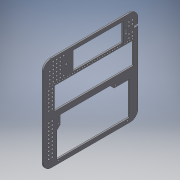
# Autodesk Inventor part: TrayPanelB
Saved by Autodesk Inventor 2017 (Build 210142000, 142)
## iProperties
Created: 2019-06-22
Part Number: TrayPanelB
Material: Generic
Document SubType Name: Modeling
Designer: DDeGo
Density: 1 g/cm^3
Appearance: Default
Author: DDeGo
Autodesk Inventor part; units mm, degrees
ref_plane "YZ Plane" through (0, 0, 0) normal (1, 0, 0) x (0, 1, 0)
ref_plane "XZ Plane" through (0, 0, 0) normal (0, 1, 0) x (-1, 0, 0)
ref_plane "XY Plane" through (0, 0, 0) normal (0, 0, 1) x (1, 0, 0)
sketch "Block1" plane through (0, 0, 0) normal (0, 0, 1) x (1, 0, 0)
  circle A0 centre (31, 19.5) radius 1.5
  line L0 (34, 5.5) -> (34, 22.5)
  line L1 (34, 22.5) -> (27, 29.5)
  line L2 (27, 29.5) -> (27, 80.5)
  circle A1 centre (31, 83.5) radius 1.5
  line L3 (134, 5.5) -> (34, 5.5)
  line L4 (173, 80.5) -> (173, 13.5)
  circle A2 centre (169, 83.5) radius 1.5
  line L5 (27, 80.5) -> (173, 80.5)
  line L6 (173, 13.5) -> (142, 13.5)
  line L7 (142, 13.5) -> (134, 5.5)
  circle A3 centre (145, 9.5) radius 1.5
  point P0 (93.25, 35.7812)
sketch "Sketch1" plane through (0, 0, 0) normal (1, 0, 0) x (0, 1, 0)
  line L0 (59.5116, 142.721) -> (59.5116, 146.221) construction
  line L1 (59.5116, 182.721) -> (159.5116, 182.721)
  line L2 (159.5116, 182.721) -> (159.5116, 142.721)
  line L3 (159.5116, 142.721) -> (158.0116, 142.721)
  line L4 (21.5116, 95.221) -> (21.5116, 139.921)
  line L5 (21.5116, 139.921) -> (180.5116, 139.921)
  line L6 (180.5116, 139.921) -> (180.5116, 95.221)
  line L7 (180.5116, 95.221) -> (21.5116, 95.221)
  line L8 (174.0116, 190.221) -> (15.0116, 190.221)
  arc A0 (15.0116, 190.221) -> (-0.4884, 174.721) centre (15.0116, 174.721) ccw
  line L9 (-0.4884, 174.721) -> (-0.4884, 15.721)
  arc A1 (-0.4884, 15.721) -> (15.0116, 0.221) centre (15.0116, 15.721) ccw
  line L10 (15.0116, 0.221) -> (174.0116, 0.221)
  arc A2 (174.0116, 0.221) -> (189.5116, 15.721) centre (174.0116, 15.721) ccw
  line L11 (189.5116, 15.721) -> (189.5116, 174.721)
  arc A3 (189.5116, 174.721) -> (174.0116, 190.221) centre (174.0116, 174.721) ccw
  line L12 (158.0116, 142.721) -> (158.0116, 146.221)
  line L13 (158.0116, 146.221) -> (59.5116, 146.221)
  line L14 (158.0116, 142.721) -> (59.5116, 142.721) construction
  line L15 (59.5116, 146.221) -> (59.5116, 182.721)
  circle A4 centre (30.5116, 69.721) radius 1.5
  line L16 (33.5116, 83.721) -> (33.5116, 66.721)
  line L17 (33.5116, 66.721) -> (26.5116, 59.721)
  line L18 (26.5116, 59.721) -> (26.5116, 8.721)
  circle A5 centre (30.5116, 5.721) radius 1.5
  line L19 (133.5116, 83.721) -> (33.5116, 83.721)
  line L20 (172.5116, 8.721) -> (172.5116, 75.721)
  circle A6 centre (168.5116, 5.721) radius 1.5
  line L21 (26.5116, 8.721) -> (172.5116, 8.721)
  line L22 (172.5116, 75.721) -> (141.5116, 75.721)
  line L23 (141.5116, 75.721) -> (133.5116, 83.721)
  circle A7 centre (144.5116, 79.721) radius 1.5
  dimension "d2" = 100
  dimension "d4" = 190
  dimension "d5" = 190
  dimension "d8" = 95
  dimension "d10" = 22
  dimension "d11" = 60
  dimension "d12" = 44.7
  dimension "d13" = 159
  dimension "d14" = 15.5
  dimension "d47" = 5.5
  dimension "d48" = 27
  dimension "d65" = 3.5
  dimension "d66" = 1.5
  dimension "d67" = 146
  dimension "d68" = 36.5
  constraints: 32 end point, 8 point on circle, 8 tangent, 4 centre point, 4 horizontal, 4 vertical, 3 equal radius, 2 perpendicular, 1 other
  measures "d2" distance between parallel lines of L0 L2
  measures "d4" distance between parallel lines of L11 L9
  measures "d5" distance between parallel lines of L8 L10
  measures "d8" distance between parallel lines of L10 L7
  measures "d10" distance between parallel lines of L4 L9
  measures "d11" distance between parallel lines of L0 L9
  measures "d12" distance between parallel lines of L5 L7
  measures "d13" distance between parallel lines of L4 L6
  measures "d14" radius of A0
  measures "d65" distance between parallel lines of L3 L13
  measures "d66" distance between parallel lines of L2 L12
  measures "d67" distance between parallel lines of L10 L13
  measures "d68" distance between parallel lines of L1 L13
extrude "Extrusion1" add sketch "Sketch1" along normal blind 2.75
sketch "Sketch2" plane through (2.75, 0, 0) normal (1, 0, 0) x (0, 0, -1)
  circle A0 centre (-148.221, 54.5116) radius 2
  line L0 (-142.721, 159.5116) -> (-142.721, 158.0116) projected
  line L1 (-146.221, 59.5116) -> (-179.9149, 59.5116) construction
  circle A1 centre (-148.221, 47.5116) radius 2
  circle A2 centre (-148.221, 40.5116) radius 2
  circle A3 centre (-148.221, 33.5116) radius 2
  circle A4 centre (-148.221, 26.5116) radius 2
  circle A5 centre (-148.221, 19.5116) radius 2
  circle A6 centre (-148.221, 12.5116) radius 2
  circle A7 centre (-155.221, 54.5116) radius 2
  circle A8 centre (-155.221, 47.5116) radius 2
  circle A9 centre (-155.221, 40.5116) radius 2
  circle A10 centre (-155.221, 33.5116) radius 2
  circle A11 centre (-155.221, 26.5116) radius 2
  circle A12 centre (-155.221, 19.5116) radius 2
  circle A13 centre (-155.221, 12.5116) radius 2
  circle A14 centre (-162.221, 54.5116) radius 2
  circle A15 centre (-162.221, 47.5116) radius 2
  circle A16 centre (-162.221, 40.5116) radius 2
  circle A17 centre (-162.221, 33.5116) radius 2
  circle A18 centre (-162.221, 26.5116) radius 2
  circle A19 centre (-162.221, 19.5116) radius 2
  circle A20 centre (-162.221, 12.5116) radius 2
  circle A21 centre (-169.221, 54.5116) radius 2
  circle A22 centre (-169.221, 47.5116) radius 2
  circle A23 centre (-169.221, 40.5116) radius 2
  circle A24 centre (-169.221, 33.5116) radius 2
  circle A25 centre (-169.221, 26.5116) radius 2
  circle A26 centre (-169.221, 19.5116) radius 2
  circle A27 centre (-169.221, 12.5116) radius 2
  circle A28 centre (-176.221, 54.5116) radius 2
  circle A29 centre (-176.221, 47.5116) radius 2
  circle A30 centre (-176.221, 40.5116) radius 2
  circle A31 centre (-176.221, 33.5116) radius 2
  circle A32 centre (-176.221, 26.5116) radius 2
  circle A33 centre (-176.221, 19.5116) radius 2
  circle A34 centre (-176.221, 12.5116) radius 2
  circle A35 centre (-183.221, 54.5116) radius 2
  circle A36 centre (-183.221, 47.5116) radius 2
  circle A37 centre (-183.221, 40.5116) radius 2
  circle A38 centre (-183.221, 33.5116) radius 2
  circle A39 centre (-183.221, 26.5116) radius 2
  circle A40 centre (-183.221, 19.5116) radius 2
  circle A41 centre (-183.221, 12.5116) radius 2
  line L2 (-148.221, 54.5116) -> (-148.221, 164.5116) construction
  circle A42 centre (-148.221, 164.5116) radius 2
  line L3 (-182.721, 159.5116) -> (-142.721, 159.5116) projected
  circle A43 centre (-148.221, 171.5116) radius 2
  circle A44 centre (-148.221, 178.5116) radius 2
  circle A45 centre (-155.221, 164.5116) radius 2
  circle A46 centre (-155.221, 171.5116) radius 2
  circle A47 centre (-155.221, 178.5116) radius 2
  circle A48 centre (-162.221, 164.5116) radius 2
  circle A49 centre (-162.221, 171.5116) radius 2
  circle A50 centre (-162.221, 178.5116) radius 2
  circle A51 centre (-169.221, 164.5116) radius 2
  circle A52 centre (-169.221, 171.5116) radius 2
  circle A53 centre (-169.221, 178.5116) radius 2
  circle A54 centre (-176.221, 164.5116) radius 2
  circle A55 centre (-176.221, 171.5116) radius 2
  circle A56 centre (-176.221, 178.5116) radius 2
  circle A57 centre (-183.221, 164.5116) radius 2
  circle A58 centre (-183.221, 171.5116) radius 2
  circle A59 centre (-183.221, 178.5116) radius 2
  circle A60 centre (-143.071, 12.5116) radius 1.5
  line L4 (-139.921, 21.5116) -> (-139.921, 180.5116) projected
  line L5 (-139.921, 12.5116) -> (-143.071, 12.5116) construction
  line L6 (-143.071, 12.5116) -> (-146.221, 12.5116) construction
  line L7 (-146.221, 12.5116) -> (-148.221, 12.5116) construction
  circle A61 centre (-143.071, 17.5419) radius 1.5
  circle A62 centre (-143.071, 22.5722) radius 1.5
  circle A63 centre (-143.071, 27.6025) radius 1.5
  circle A64 centre (-143.071, 32.6328) radius 1.5
  circle A65 centre (-143.071, 37.6631) radius 1.5
  circle A66 centre (-143.071, 42.6934) radius 1.5
  circle A67 centre (-143.071, 47.7237) radius 1.5
  circle A68 centre (-143.071, 52.754) radius 1.5
  circle A69 centre (-143.071, 57.7843) radius 1.5
  circle A70 centre (-143.071, 62.8146) radius 1.5
  circle A71 centre (-143.071, 67.8449) radius 1.5
  circle A72 centre (-143.071, 72.8752) radius 1.5
  circle A73 centre (-143.071, 77.9055) radius 1.5
  circle A74 centre (-143.071, 82.9358) radius 1.5
  circle A75 centre (-143.071, 87.9661) radius 1.5
  circle A76 centre (-143.071, 92.9964) radius 1.5
  circle A77 centre (-143.071, 98.0267) radius 1.5
  circle A78 centre (-143.071, 103.057) radius 1.5
  circle A79 centre (-143.071, 108.0873) radius 1.5
  circle A80 centre (-143.071, 113.1176) radius 1.5
  circle A81 centre (-143.071, 118.1479) radius 1.5
  circle A82 centre (-143.071, 123.1782) radius 1.5
  circle A83 centre (-143.071, 128.2085) radius 1.5
  circle A84 centre (-143.071, 133.2388) radius 1.5
  circle A85 centre (-143.071, 138.2691) radius 1.5
  circle A86 centre (-143.071, 143.2994) radius 1.5
  circle A87 centre (-143.071, 148.3298) radius 1.5
  circle A88 centre (-143.071, 153.3601) radius 1.5
  circle A89 centre (-143.071, 158.3904) radius 1.5
  circle A90 centre (-143.071, 163.4207) radius 1.5
  circle A91 centre (-143.071, 168.451) radius 1.5
  circle A92 centre (-143.071, 173.4813) radius 1.5
  circle A93 centre (-143.071, 178.5116) radius 1.5
  line L8 (-148.221, 178.5116) -> (-143.071, 178.5116) construction
  line L9 (-146.221, 59.5116) -> (-182.721, 59.5116) construction
  line L10 (-146.221, 158.0116) -> (-146.221, 59.5116) projected
  circle A94 centre (-136.771, 10.5116) radius 2
  line L11 (-139.921, 12.5116) -> (-136.771, 12.5116) construction
  line L12 (-136.771, 12.5116) -> (-136.771, 10.5116) construction
  circle A95 centre (-136.771, 17.5116) radius 2
  circle A96 centre (-129.771, 10.5116) radius 2
  circle A97 centre (-129.771, 17.5116) radius 2
  circle A98 centre (-122.771, 10.5116) radius 2
  circle A99 centre (-122.771, 17.5116) radius 2
  circle A100 centre (-115.771, 10.5116) radius 2
  circle A101 centre (-115.771, 17.5116) radius 2
  circle A102 centre (-108.771, 10.5116) radius 2
  circle A103 centre (-108.771, 17.5116) radius 2
  circle A104 centre (-101.771, 10.5116) radius 2
  circle A105 centre (-101.771, 17.5116) radius 2
  circle A106 centre (-94.771, 10.5116) radius 2
  circle A107 centre (-94.771, 17.5116) radius 2
  circle A108 centre (-87.771, 10.5116) radius 2
  circle A109 centre (-87.771, 17.5116) radius 2
  circle A110 centre (-80.771, 10.5116) radius 2
  circle A111 centre (-80.771, 17.5116) radius 2
  circle A112 centre (-73.771, 10.5116) radius 2
  circle A113 centre (-73.771, 17.5116) radius 2
  circle A114 centre (-66.771, 10.5116) radius 2
  circle A115 centre (-66.771, 17.5116) radius 2
  circle A116 centre (-59.771, 10.5116) radius 2
  circle A117 centre (-59.771, 17.5116) radius 2
  circle A118 centre (-52.771, 10.5116) radius 2
  circle A119 centre (-52.771, 17.5116) radius 2
  circle A120 centre (-45.771, 10.5116) radius 2
  circle A121 centre (-45.771, 17.5116) radius 2
  circle A122 centre (-38.771, 10.5116) radius 2
  circle A123 centre (-38.771, 17.5116) radius 2
  circle A124 centre (-31.771, 10.5116) radius 2
  circle A125 centre (-31.771, 17.5116) radius 2
  circle A126 centre (-24.771, 10.5116) radius 2
  circle A127 centre (-24.771, 17.5116) radius 2
  circle A128 centre (-17.771, 10.5116) radius 2
  circle A129 centre (-17.771, 17.5116) radius 2
  point P0 (0, 0)
  dimension "d15" = 4
  dimension "d17" = 5
  dimension "d20" = 7
  dimension "d23" = 7
  dimension "d28" = 5
  dimension "d31" = 7
  dimension "d34" = 7
  dimension "d37" = 3
  dimension "d40" = 5.0303
  dimension "d69" = 2
  dimension "d77" = 7
  dimension "d80" = 7
  dimension "d83" = 2
  constraints: 129 centre point, 16 end point, 9 horizontal, 8 equal radius, 8 vertical alignment, 3 vertical, 2 collinear, 2 point on line, 1 coincident, 1 horizontal alignment, 1 perpendicular, 241 other
  measures "d15" diameter of A0
  measures "d17" distance from line of L2.start L1
  measures "d20" distance of L2.start A1.centre
  measures "d23" distance of L2.start A7.centre
  measures "d28" distance from line of L3 A42.centre
  measures "d31" distance of A42.centre A43.centre
  measures "d34" distance of A42.centre A45.centre
  measures "d37" diameter of A60
  measures "d40" distance of L5.end A61.centre
  measures "d69" distance between parallel lines of L10 L2
  measures "d77" distance of L12.end A95.centre
  measures "d80" distance of L12.end A96.centre
  measures "d83" distance of L11.end L12.end
extrude "Extrusion2" cut sketch "Sketch2" against normal blind 10 contours A3 | A4 | A5 | A6 | A10 | A11 | A12 | A13 | A17 | A18 | A19 | A20 | A24 | A25 | A26 | A27 | A31 | A32 | A33 | A38 | A39 | A40 | A43 | A44 | A46 | A47 | A52 | A53 | A55 | A56 | A60 | A61 | A62 | A63 | A64 | A65 | A66 | A67 | A68 | A69 | A70 | A71 | A72 | A73 | A74 | A75 | A76 | A77 | A78 | A79 | A80 | A81 | A82 | A83 | A84 | A85 | A86 | A87 | A88 | A90 | A91 | A92 | A93 | A94 | A95 | A96 | A97 | A98 | A99 | A100 | A101 | A102 | A103 | A104 | A105 | A110 | A111 | A112 | A113 | A114 | A115 | A116 | A117 | A118 | A119 | A120 | A121 | A122 | A123 | A124 | A125 | A126 | A127 | A128 | A129
sketch "Sketch3" plane through (0, 0, 0) normal (-1, 0, 0) x (0, 0, 1)
  line L0 (167.221, 168.2116) -> (157.221, 168.2116)
  line L1 (157.221, 168.2116) -> (157.221, 163.9116)
  line L2 (157.221, 163.9116) -> (167.221, 163.9116)
  line L3 (167.221, 163.9116) -> (167.221, 168.2116)
  line L4 (142.721, 158.0116) -> (142.721, 159.5116) projected
  line L5 (142.721, 159.5116) -> (182.721, 159.5116) projected
  line L6 (164.371, 189.5116) -> (160.071, 189.5116)
  line L7 (160.071, 189.5116) -> (160.071, 181.5116)
  line L8 (160.071, 181.5116) -> (164.371, 181.5116)
  line L9 (164.371, 181.5116) -> (164.371, 189.5116)
  line L10 (174.721, 189.5116) -> (15.721, 189.5116) projected
  line L11 (162.221, 181.5116) -> (162.221, 168.2116) construction
  point P0 (0, 0)
  point P1 (143.721, 59.5116)
  dimension "d49" = 4.3
  dimension "d50" = 10
  dimension "d51" = 14.5
  dimension "d52" = 4.4
  dimension "d55" = 4.3
  dimension "d56" = 8
  constraints: 18 end point, 4 parallel, 2 horizontal, 2 midpoint, 2 perpendicular, 1 point on line, 1 vertical, 1 other
  measures "d49" distance of L2.end L0.start
  measures "d50" distance of L1.end L2.end
  measures "d52" distance between parallel lines of L5 L2
  measures "d55" distance of L7.end L8.end
  measures "d56" distance between parallel lines of L6 L8
extrude "Extrusion3" cut sketch "Sketch3" against normal blind 10
sketch "Sketch4" plane through (0, 0, 0) normal (-1, 0, 0) x (0, 0, 1)
  circle A0 centre (179.721, 179.0116) radius 2.05
  line L0 (190.221, 15.0116) -> (190.221, 174.0116) projected
  line L1 (174.721, 189.5116) -> (164.371, 189.5116) projected
  circle A1 centre (10.721, 10.0116) radius 2.05
  line L2 (15.721, -0.4884) -> (174.721, -0.4884) projected
  line L3 (0.221, 174.0116) -> (0.221, 15.0116) projected
  line L4 (179.721, 179.0116) -> (10.721, 179.0116) construction
  line L5 (10.721, 179.0116) -> (10.721, 10.0116) construction
  line L6 (10.721, 10.0116) -> (179.721, 10.0116) construction
  line L7 (179.721, 10.0116) -> (179.721, 179.0116) construction
  circle A2 centre (10.721, 179.0116) radius 2.05
  circle A3 centre (179.721, 10.0116) radius 2.05
  point P0 (0, 0)
  dimension "d57" = 10.5
  dimension "d58" = 10.5
  dimension "d59" = 4.1
  dimension "d60" = 10.5
  dimension "d61" = 10.5
  dimension "d62" = 4.1
  constraints: 8 end point, 4 centre point, 2 coincident, 2 equal radius, 2 parallel, 1 horizontal, 1 perpendicular
  measures "d57" distance from line of L0 L4.start
  measures "d58" distance from line of L1 L4.start
  measures "d59" diameter of A0
  measures "d60" distance from line of L2 L5.end
  measures "d61" distance from line of L3 L5.end
  measures "d62" diameter of A1
extrude "Extrusion4" [suppressed]
sketch "Sketch5" plane through (2.75, 0, 0) normal (1, 0, 0) x (0, 0, -1)
  circle A0 centre (-165.721, 45.5116) radius 2
  line L0 (-182.721, 59.5116) -> (-182.721, 159.5116) projected
  line L1 (-146.221, 59.5116) -> (-182.721, 59.5116) projected
  point P0 (0, 0)
  dimension "d70" = 17
  dimension "d71" = 14
  dimension "d72" = 4
  constraints: 1 centre point
  measures "d70" distance from line of L0 A0.centre
  measures "d71" distance from line of A0.centre L1
  measures "d72" diameter of A0
extrude "Extrusion5" cut sketch "Sketch5" against normal blind 10
body "Solid1"
